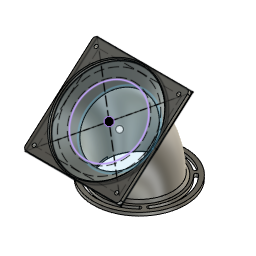
120-80-Tilted-FanAdaptor (Autodesk Fusion 360 design; units mm, degrees)
Autodesk Fusion 360 part; units mm, degrees
sketch "Sketch1" plane through (0, 0, 0) normal (0, 0, 1) x (1, 0, 0) in component "Component"
  circle A0 centre (0, 0) radius 40
  line L0 (35.75, -35.75) -> (-35.75, -35.75) construction
  line L1 (-35.75, -35.75) -> (-35.75, 35.75) construction
  line L2 (-35.75, 35.75) -> (35.75, 35.75) construction
  line L3 (35.75, 35.75) -> (35.75, -35.75) construction
  line L4 (35.75, -35.75) -> (-35.75, 35.75) construction
  line L5 (-35.75, -35.75) -> (35.75, 35.75) construction
  circle A1 centre (0, 0) radius 57.9733
  arc A2 (30.2895, 43.2579) -> (-37.341, 37.341) centre (0, 0) ccw
  arc A3 (27.7084, 39.5717) -> (30.2895, 43.2579) centre (28.999, 41.4148) ccw
  arc A4 (27.7084, 39.5717) -> (-34.159, 34.159) centre (0, 0) ccw
  arc A5 (-37.341, 37.341) -> (-34.159, 34.159) centre (-35.75, 35.75) ccw
  arc A6 (28.999, 41.4148) -> (-35.75, 35.75) centre (0, 0) ccw construction
  arc A7 (43.2579, -30.2895) -> (37.341, 37.341) centre (0, 0) ccw
  arc A8 (39.5717, -27.7084) -> (43.2579, -30.2895) centre (41.4148, -28.999) ccw
  arc A9 (39.5717, -27.7084) -> (34.159, 34.159) centre (0, 0) ccw
  arc A10 (37.341, 37.341) -> (34.159, 34.159) centre (35.75, 35.75) ccw
  arc A11 (41.4148, -28.999) -> (35.75, 35.75) centre (0, 0) ccw construction
  arc A12 (-30.2895, -43.2579) -> (37.341, -37.341) centre (0, 0) ccw
  arc A13 (-27.7084, -39.5717) -> (-30.2895, -43.2579) centre (-28.999, -41.4148) ccw
  arc A14 (-27.7084, -39.5717) -> (34.159, -34.159) centre (0, 0) ccw
  arc A15 (37.341, -37.341) -> (34.159, -34.159) centre (35.75, -35.75) ccw
  arc A16 (-28.999, -41.4148) -> (35.75, -35.75) centre (0, 0) ccw construction
  arc A17 (-43.2579, 30.2895) -> (-37.341, -37.341) centre (0, 0) ccw
  arc A18 (-39.5717, 27.7084) -> (-43.2579, 30.2895) centre (-41.4148, 28.999) ccw
  arc A19 (-39.5717, 27.7084) -> (-34.159, -34.159) centre (0, 0) ccw
  arc A20 (-37.341, -37.341) -> (-34.159, -34.159) centre (-35.75, -35.75) ccw
  arc A21 (-41.4148, 28.999) -> (-35.75, -35.75) centre (0, 0) ccw construction
  line L6 (0, 0) -> (-41.4148, 28.999) construction
  line L7 (0, 0) -> (-35.75, -35.75) construction
  dimension "d1" = 80
  dimension "d2" = 71.5
  dimension "d3" = 71.5
  dimension "d35" = 80
  dimension "d49" = 115.9466
  constraint coincident A0.centre A1.centre
  constraint perpendicular L0 L1
  constraint parallel L0 L2
  constraint parallel L1 L3
  constraint horizontal L0
  constraint coincident L4 A0.centre
  constraint coincident L5 A0.centre
  constraint tangent A2 A3
  constraint tangent A3 A4
  constraint tangent A4 A5
  constraint tangent A2 A5
  constraint coincident L1.end L2.start
  constraint tangent A7 A8
  constraint tangent A8 A9
  constraint tangent A9 A10
  constraint tangent A7 A10
  constraint coincident L2.end L3.start
  constraint tangent A12 A13
  constraint tangent A13 A14
  constraint tangent A14 A15
  constraint tangent A12 A15
  constraint coincident L0.start L3.end
  constraint tangent A17 A18
  constraint tangent A18 A19
  constraint tangent A19 A20
  constraint tangent A17 A20
  constraint coincident L0.end L1.start
  measures "d1" diameter of A0
  measures "d2" distance of L1.end L2.end
  measures "d3" distance of L0.end L1.end
  measures "d35" angle of L6 L7
  measures "d49" diameter of A1
extrude "Extrude1" add sketch "Sketch1" along normal blind 4 makes body 1 in component "Component"
sketch "Sketch2" plane through (0, 0, 0) normal (1, 0, 0) x (0, 1, 0) in component "Component"
  arc A0 (0, 0) -> (-22.0077, 44.0058) centre (-55, 0) ccw
  arc A1 (0, 0) -> (-24.87, 66.0491) centre (-100.1407, 0) ccw
  constraint coincident A0.start A1.start
pipe "Pipe1" add diameter 84 wall 2 path "Sketch2" along A1 bodies 1 in component "Component"
sketch "Sketch5" plane through (0, -43.5635, 49.6458) normal (0, -0.659563, 0.751649) x (1, 0, 0) in component "Component"
  circle A0 centre (0, 24.87) radius 40
  circle A1 centre (0, 24.87) radius 42
  circle A2 centre (0, 24.87) radius 42
  constraint concentric A0 A2
ref_plane "WorkPlane1" through (0, -38.0613, 81.0821) normal (0, -0.659563, 0.751649) x (1, 0, 0) in component "Component"
sketch "Sketch3" plane through (0, -38.0613, 81.0821) normal (0, -0.659563, 0.751649) x (1, 0, 0) in component "Component"
  circle A0 centre (0, 0) radius 40
  circle A1 centre (0, 0) radius 42 construction
  circle A2 centre (0, 0) radius 60
  circle A3 centre (0, 0) radius 52 construction
  line L0 (52, -52) -> (-52, -52) construction
  line L1 (-52, -52) -> (-52, 52) construction
  line L2 (-52, 52) -> (52, 52) construction
  line L3 (52, 52) -> (52, -52) construction
  line L4 (52, -52) -> (-52, 52) construction
  line L5 (-52, -52) -> (52, 52) construction
  line L6 (60, 60) -> (-60, 60)
  line L7 (-60, 60) -> (-60, -60)
  line L8 (-60, -60) -> (60, -60)
  line L9 (60, -60) -> (60, 60)
  line L10 (60, 60) -> (-60, -60) construction
  line L11 (-60, 60) -> (60, -60) construction
  circle A4 centre (0, 0) radius 58
  dimension "d11" = 120
  dimension "d12" = 104
  dimension "d13" = 104
  dimension "d14" = 104
  dimension "d15" = 120
  dimension "d16" = 120
  dimension "d24" = 116
  constraint concentric A0 A2
  constraint coincident A0.centre A1.centre
  constraint perpendicular L0 L1
  constraint parallel L0 L2
  constraint parallel L1 L3
  constraint horizontal L0
  constraint coincident L4 A0.centre
  constraint coincident L5 A0.centre
  constraint perpendicular L6 L7
  constraint parallel L6 L8
  constraint parallel L7 L9
  constraint horizontal L6
  constraint coincident L10 A0.centre
  constraint coincident L11 A0.centre
  measures "d11" diameter of A2
  measures "d12" diameter of A3
  measures "d13" distance of L1.end L2.end
  measures "d14" distance of L0.end L1.end
  measures "d15" distance of L7.end L8.end
  measures "d16" distance of L6.end L7.end
  measures "d24" diameter of A4
loft "Loft1" add profiles "Sketch5", "Sketch3" section 1 section 2 contours A2 | A2 L8 L9 | A2 L6 L9 | A2 L6 L7 | A2 L7 L8 separate body makes body 2 in component "Component"
loft "Loft2" cut profiles "Sketch5", "Sketch3" section 1 contours A0 section 2 contours A4 bodies 2 in component "Component"
extrude "Extrude3" add sketch "Sketch3" along normal blind 5 contours A2 | A2 L8 L9 | A2 L6 L9 | A2 L6 L7 | A2 L7 L8 bodies 2 in component "Component"
sketch "Sketch6" plane through (0, -60.0526, 68.437) normal (0, -0.659563, 0.751649) x (1, 0, 0) in component "Component"
  circle A0 centre (0, 24.87) radius 58
  line L0 (60, -35.13) -> (60, 84.87)
  line L1 (60, 84.87) -> (-60, 84.87)
  line L2 (-60, 84.87) -> (-60, -35.13)
  line L3 (-60, -35.13) -> (60, -35.13)
  circle A1 centre (52, -27.13) radius 2.1
  circle A2 centre (-52, -27.13) radius 2.1
  circle A3 centre (-52, 76.87) radius 2.1
  circle A4 centre (52, 76.87) radius 2.1
  point P0 (-52, 76.87)
  point P1 (52, 76.87)
  point P2 (52, -27.13)
  point P3 (-52, -27.13)
  dimension "d27" = 4.2
  dimension "d28" = 4.2
  dimension "d29" = 4.2
  dimension "d30" = 4.2
  constraint coincident P2 A1.centre
  constraint coincident P3 A2.centre
  constraint coincident P0 A3.centre
  constraint coincident P1 A4.centre
  measures "d27" diameter of A1
  measures "d28" diameter of A2
  measures "d29" diameter of A3
  measures "d30" diameter of A4
extrude "Extrude4" cut sketch "Sketch6" against normal blind 12 contours A1 | A2 | A3 | A4 bodies 2 in component "Component"
fillet "Fillet1" radius 4 4 edges at (-60, -84.8091, 43.3874) (-60, 5.3888, 122.535) (60, -84.8091, 43.3874) (60, 5.3888, 122.535) on bodies 2 in component "Component"
chamfer "Chamfer2" distance 1.5 angle 45 2 edges at (0, 40, 0) (0, -40, 0) on bodies 1 in component "Component"
chamfer "Chamfer3" distance 3 angle 45 1 edges at (0, -42.1378, 4) on bodies 1 in component "Component"
chamfer "Chamfer4" distance 1.2 angle 45 1 edges at (-54.075, -25.5942, 98.6738) on bodies 2 in component "Component"
sketch "Sketch2 (2)" plane through (0, 0, 0) normal (0, 1, 0) x (1, 0, 0)
sketch "Sketch3 (2)" plane through (0, -38.0613, 81.0821) normal (0, -0.659563, 0.751649) x (1, 0, 0)
  line L0 (-53.1789, -42.1656) -> (-44.2354, -42.1656)
  line L1 (-44.2354, -42.1656) -> (-44.2354, -22.5853)
  line L2 (-44.2354, -22.5853) -> (-53.1789, -22.5853)
  line L3 (-53.1789, -22.5853) -> (-53.1789, -42.1656)
  constraint horizontal L0
  constraint vertical L1
  constraint horizontal L2
  constraint vertical L3
component "Component" placed x (1, 0, 0) y (0, 1, 0) z (0, 0, 1) at (0, 0, 0)
equation "d13 = Fan120ScrewHoleDistance"
equation "d14 = Fan120ScrewHoleDistance"
equation "d15 = fanSize"
equation "d16 = fanSize"
equation "fanScrewHoleSize = 4.2 mm"
equation "Fan120ScrewHoleDistance = 104 mm"
equation "fanSize = 120 mm"
equation "d27 = fanScrewHoleSize"
equation "d28 = fanScrewHoleSize"
equation "d29 = fanScrewHoleSize"
equation "d30 = fanScrewHoleSize"
equation "slotSize = 4.5 mm"
